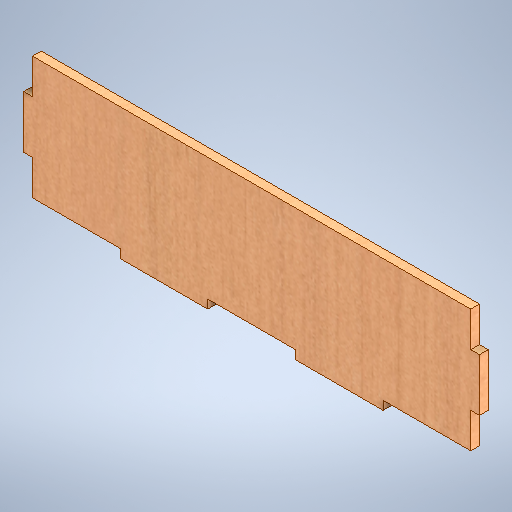
# Autodesk Inventor part: Lat1(3)
Saved by Autodesk Inventor 2025 (Build 290162000, 162)
## iProperties
Created: 2024-11-02
Part Number: Lat1(3)
Material: Wood (Cherry)
Document SubType Name: Sheet Metal
Designer: g.marin
Density: 0.63 g/cm^3
Sheet Metal Rule: Default
Appearance: Cherry - Natural Low Gloss
Author: g.marin
Autodesk Inventor part; units mm, degrees
ref_plane "YZ Plane" through (0, 0, 0) normal (1, 0, 0) x (0, 1, 0)
ref_plane "XZ Plane" through (0, 0, 0) normal (0, 1, 0) x (-1, 0, 0)
ref_plane "XY Plane" through (0, 0, 0) normal (0, 0, 1) x (1, 0, 0)
sketch "Sketch1" plane through (0, 0, 0) normal (0, 0, 1) x (1, 0, 0)
  line L0 (-130, -35) -> (130, -35)
  line L1 (130, -35) -> (130, 35)
  line L2 (130, 35) -> (-130, 35)
  line L3 (-130, 35) -> (-130, -35)
  line L4 (-130, -35) -> (130, 35) construction
  line L5 (130, -35) -> (-130, 35) construction
  line L6 (-75, -35) -> (-25, -35)
  line L7 (-25, -35) -> (-25, -40)
  line L8 (-25, -40) -> (-75, -40)
  line L9 (-75, -40) -> (-75, -35)
  line L10 (25, -35) -> (75, -35)
  line L11 (75, -35) -> (75, -40)
  line L12 (75, -40) -> (25, -40)
  line L13 (25, -40) -> (25, -35)
  line L14 (130, 35) -> (125, 35)
  line L15 (125, 35) -> (125, 15)
  line L16 (125, 15) -> (130, 15)
  line L17 (130, 15) -> (130, 35)
  line L18 (130, -35) -> (125, -35)
  line L19 (125, -35) -> (125, -15)
  line L20 (125, -15) -> (130, -15)
  line L21 (130, -15) -> (130, -35)
  line L22 (0, 35) -> (0, -35) construction
  line L23 (-125, 35) -> (-125, 15)
  line L24 (-125, 15) -> (-130, 15)
  line L25 (-125, -35) -> (-125, -15)
  line L26 (-125, -15) -> (-130, -15)
  point P0 (0, 0)
  point P1 (-75, -37.5)
  point P2 (-130, -15)
  point P3 (130, -15)
  point P4 (130, 15)
  dimension "d0" = 260
  dimension "d1" = 70
  dimension "d2" = 50
  dimension "d3" = 50
  dimension "d4" = 50
  dimension "d5" = 55
  dimension "d6" = 5
  dimension "d9" = 30
  dimension "d10" = 20
  dimension "d12" = 5
  constraints: 54 end point, 10 parallel, 6 symmetric about line, 5 horizontal, 5 midpoint, 5 perpendicular, 5 point on line
  measures "d0" distance of L1.end L2.end
  measures "d1" distance of L0.end L1.end
  measures "d2" distance of L7.end L8.end
  measures "d3" distance of L11.end L12.end
  measures "d4" distance between parallel lines of L13 L7
  measures "d5" horizontal distance of point (-75, -37.5) L0.start
  measures "d6" distance of L6.end L7.end
  measures "d9" distance of L19.end L15.end
  measures "d10" distance of L18.end L19.end
  measures "d12" distance of L15.end L16.end
extrude "Extrusion1" add sketch "Sketch1" along normal blind 5 contours L25 L26 L3 L24 L23 L2 L15 L16 L1 L20 L19 L0 | L0 L7 L8 L9 | L0 L11 L12 L13
equation "\"BendRadius\" = Thickness"
equation "\"BendReliefWidth\" = Thickness"
equation "\"BendReliefDepth\" = 0.5 * Thickness"
equation "\"CornerReliefSize\" = 4 * Thickness"
equation "\"MinimumRemnant\" = 2 * Thickness"
equation "\"TransitionRadius\" = BendRadius"
equation "\"JacobiRadiusSize\" = BendRadius"
equation "\"GapSize\" = Thickness"
equation "\"Thickness\" = 3.048"
body "Solid1"
